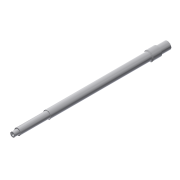
# Autodesk Inventor part: PP-09
Saved by Autodesk Inventor 2022 (Build 260148000, 148)
## iProperties
Created: 2008-09-23
Part Number: PP-09
Document SubType Name: Modeling
Designer: Mark Flayler
Mass: 0.807317 g
Surface Area: 27.0821 cm^2
Volume: 0.76162 cm^3
Density: 1.06 g/cm^3
Material: ABS Plastic
Description: SHAFT
Appearance: Smooth - White
Author: Mark Flayler
Autodesk Inventor part; units mm, degrees
ref_plane "YZ Plane" through (0, 0, 0) normal (1, 0, 0) x (0, 1, 0)
ref_plane "XZ Plane" through (0, 0, 0) normal (0, 1, 0) x (-1, 0, 0)
ref_plane "XY Plane" through (0, 0, 0) normal (0, 0, 1) x (1, 0, 0)
sketch "Sketch1" plane through (0, 0, 0) normal (0, 0, 1) x (1, 0, 0)
  line L0 (0, 0) -> (0, 99.2)
  line L1 (0.9, 0) -> (1.5, 0)
  line L2 (1.5, 0) -> (1.5, 3.2)
  line L3 (1.5, 3.2) -> (2.1, 3.2)
  line L4 (2.1, 3.2) -> (2.1, 22.1)
  line L5 (2.1, 22.1) -> (2.5, 22.1)
  line L6 (2.5, 22.1) -> (2.5, 86.7)
  line L7 (2.5, 86.7) -> (3.1, 87.3)
  line L8 (3.1, 87.3) -> (3.1, 92.7)
  line L9 (3.1, 92.7) -> (2.5, 92.7)
  line L10 (2.5, 92.7) -> (2.5, 99.2)
  line L11 (2.5, 99.2) -> (2.075, 99.2)
  line L12 (2.075, 99.2) -> (2.075, 92.7)
  line L13 (2.075, 92.7) -> (1.9, 92.3)
  line L14 (1.9, 92.3) -> (1.9, 5.2)
  line L15 (1.9, 5.2) -> (0.9, 5.2)
  line L16 (0.9, 5.2) -> (0.9, 0)
  dimension "d0" = 45
  dimension "d1" = 99.2
  dimension "d2" = 92.7
  dimension "d3" = 86.7
  dimension "d4" = 22.1
  dimension "d5" = 3.2
  dimension "d6" = 1.8
  dimension "d7" = 3
  dimension "d8" = 4.2
  dimension "d9" = 5.2
  dimension "d10" = 3.8
  dimension "d11" = 4.15
  dimension "d12" = 5
  dimension "d13" = 6.2
  dimension "d14" = 92.3
  dimension "d15" = 5
  constraints: 34 end point, 9 parallel, 5 perpendicular, 3 horizontal alignment, 1 vertical
  measures "d0" angle of L6 L7
  measures "d1" distance of L0.start L0.end
  measures "d2" distance from line of L0.start L9
  measures "d3" vertical distance of L0.start L6.end
  measures "d4" distance from line of L5 L0.start
  measures "d5" distance between parallel lines of L1 L3
  measures "d6" diameter of L16 L0
  measures "d7" diameter of L2 L0
  measures "d8" diameter of L4 L0
  measures "d9" distance from line of L0.start L15
  measures "d10" diameter of L14 L0
  measures "d11" diameter of L12 L0
  measures "d12" diameter of L10 L0
  measures "d13" diameter of L8 L0
  measures "d14" vertical distance of L13.end L0.start
  measures "d15" diameter of L6 L0
revolve "Revolution1" add sketch "Sketch1" angle 360 about axis through (0, 0, 0) along (0, 1, 0)
sketch "Sketch2" plane through (0, 0, 0) normal (0, 0, 1) x (1, 0, 0)
  line L0 (-0.9, 0) -> (0.9, 0) projected
  line L1 (-4, 96) -> (0, 96) construction
  line L2 (0, -19.84) -> (0, 119.04) projected
  line L3 (0, 96) -> (-8, 96)
  line L4 (-8, 96) -> (-8, 99.2)
  line L5 (-8, 99.2) -> (0, 99.2)
  line L6 (0, 99.2) -> (0, 96)
  line L7 (-2.075, 99.2) -> (2.075, 99.2) projected
  dimension "d17" = 96
  dimension "d18" = 4
  dimension "d19" = 8
  constraints: 10 end point, 3 parallel, 1 collinear, 1 horizontal, 1 perpendicular, 1 point on line
  measures "d17" distance between parallel lines of L1 L0
  measures "d18" distance of L1.start L1.end
  measures "d19" distance between parallel lines of L4 L2
extrude "Extrusion1" cut sketch "Sketch2" against normal mid plane 2
body "Solid1"
